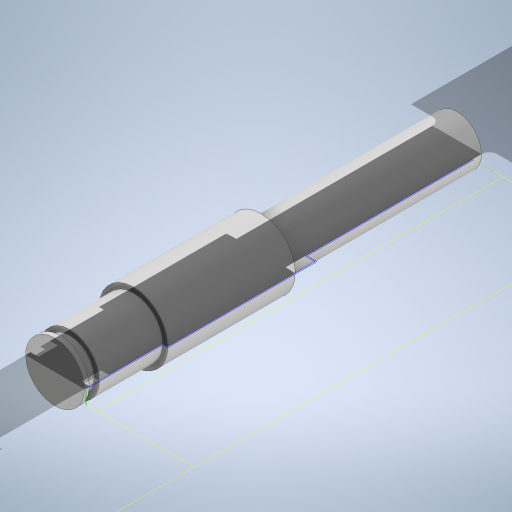
# Autodesk Inventor part: eje
Saved by Autodesk Inventor 2023.1 (Build 271208000, 208)
## iProperties
Created: 2022-08-05
Part Number: eje
Material: Genérico
Document SubType Name: Modeling
Designer: Lab. de Manufactura
Density: 1 g/cm^3
Appearance: Valor por defecto
Author: Lab. de Manufactura
Autodesk Inventor part; units mm, degrees
ref_plane "YZ Plane" through (0, 0, 0) normal (1, 0, 0) x (0, 1, 0)
ref_plane "XZ Plane" through (0, 0, 0) normal (0, 1, 0) x (-1, 0, 0)
ref_plane "XY Plane" through (0, 0, 0) normal (0, 0, 1) x (1, 0, 0)
sketch "Boceto1" plane through (0, 0, 0) normal (1, 0, 0) x (0, 1, 0)
  line L0 (0, 0) -> (3, 0)
  line L1 (3, 0) -> (3, -0.5)
  line L2 (3.5, -21) -> (6.5, -21)
  line L3 (6.5, -21) -> (6.5, -21)
  line L4 (6.5, -21) -> (2.5, -21)
  line L5 (2.5, -21) -> (2.5, -41)
  line L6 (0, 0) -> (0, -41)
  line L7 (2.5, -41) -> (0, -41)
  line L8 (3, -8) -> (3.5, -8)
  line L9 (3.5, -8) -> (3.5, -21)
  line L10 (3, -8) -> (3, -11.9913) construction
  line L11 (3, -0.5) -> (2.5, -0.5)
  line L12 (2.5, -0.5) -> (2.5, -1.5)
  line L13 (2.5, -1.5) -> (3, -1.5)
  line L14 (3, -1.5) -> (3, -0.5) construction
  line L15 (3, -0.5) -> (3, -1.5)
  line L16 (3, -1.5) -> (3, -8)
  point P0 (3.5, -14.5)
  dimension "d0" = 3
  dimension "d3" = 20
  dimension "d4" = 0
  dimension "d5" = 2.5
  dimension "d8" = 13
  dimension "d9" = 0.5
  dimension "d10" = 3
  dimension "d11" = 8
  dimension "d12" = 6.5
  dimension "d13" = 0.5
  dimension "d14" = 1
  constraints: 34 end point, 9 perpendicular, 4 horizontal, 4 vertical, 3 parallel, 2 midpoint
  measures "d0" distance of L0.start L0.end
  measures "d3" distance of L4.end L5.end
  measures "d4" distance of L2.end L3.end
  measures "d5" distance from line of L0.start L5
  measures "d8" distance of L2.start L8.end
  measures "d9" distance from line of L1 point (3.5, -14.5)
  measures "d10" distance from line of point (6.5, -21) L9
  measures "d11" distance of L0.end L8.start
  measures "d12" distance between parallel lines of L8 L13
  measures "d13" distance between parallel lines of L1 L12
  measures "d14" distance of L11.end L12.end
revolve "Revolución2" add sketch "Boceto1" angle 360 about axis through (0, 0, 0) along (0, 0, -1) contours L0 L1 L11 L12 L13 L16 L8 L9 L4 L5 L7 L6
